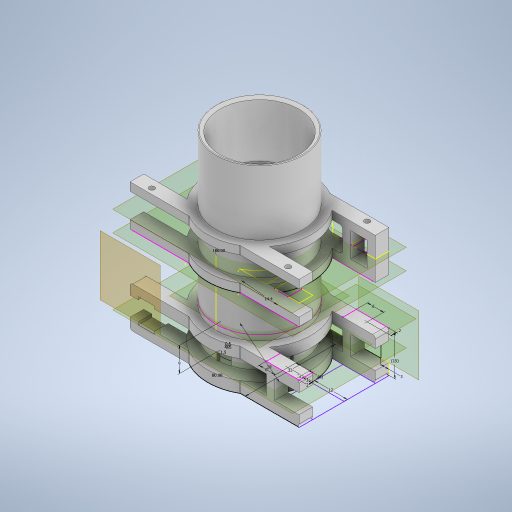
# Autodesk Inventor part: 다단로켓벨브1_ver3
Saved by Autodesk Inventor 2023 (Build 270158000, 158)
## iProperties
Created: 2023-08-24
Part Number: 다단로켓벨브1_ver3
Material: 일반
Document SubType Name: Modeling
Designer: rlatk
Density: 1 g/cm^3
Appearance: 기본값
Author: rlatk
Autodesk Inventor part; units mm, degrees
ref_plane "YZ Plane" through (0, 0, 0) normal (1, 0, 0) x (0, 1, 0)
ref_plane "XZ Plane" through (0, 0, 0) normal (0, 1, 0) x (-1, 0, 0)
ref_plane "XY Plane" through (0, 0, 0) normal (0, 0, 1) x (1, 0, 0)
sketch "스케치1" plane through (0, 0, 0) normal (0, 1, 0) x (-1, 0, 0)
  circle A0 centre (0, 0) radius 14
  circle A1 centre (0, 0) radius 16
  circle A2 centre (0, 0) radius 19
  line L0 (-9.4207, 16.5) -> (-9.4207, -16.5)
  line L1 (-19, 0) -> (-31, 0)
  line L2 (-9.4207, 16.5) -> (-31, 16.5)
  line L3 (-31, 11.5) -> (-9.4207, 11.5)
  line L4 (-9.4207, 11.5) -> (-9.4207, 16.5)
  line L5 (-9.4207, -16.5) -> (-31, -16.5)
  line L6 (-31, -11.5) -> (-9.4207, -11.5)
  line L7 (-31, 0) -> (-31, 16.5)
  line L8 (-31, 0) -> (-31, -16.5)
  line L9 (-19, -16.5) -> (-19, 16.5)
  point P0 (-15.1245, -11.5)
  point P1 (-15.1245, 11.5)
  point P2 (-9.4207, -11.5)
  point P3 (-9.4207, 11.5)
  point P4 (-19, 11.5)
  point P5 (-19, -11.5)
  dimension "d0" = 28
  dimension "d1" = 2
  dimension "d26" = 3
  dimension "d51" = 33
  dimension "d53" = 12
  constraints: 20 end point, 5 point on line, 3 centre point, 3 point on circle, 2 horizontal, 2 perpendicular, 1 coincident, 1 parallel, 1 symmetric about line, 1 vertical
  measures "d0" diameter of A0
  measures "d1" radial gap between concentric circles of A0 A1
  measures "d26" radial gap between concentric circles of A1 A2
  measures "d51" distance of L0.start L0.end
  measures "d53" distance of L1.start L1.end
extrude "돌출1" add sketch "스케치1" along normal blind 39 contours A0 L0 A1 | A0 L0 L6 A1 L3 | L3 A1 L0 | L0 A1 L6
sketch "스케치2" plane through (0, 0, 0) normal (0, 1, 0) x (-1, 0, 0)
  point P0 (0, 0)
ref_plane "작업 평면1" through (0, 18, 0) normal (0, -1, 0) x (1, 0, 0)
sketch "스케치3" plane through (0, 39, 0) normal (0, 1, 0) x (1, 0, 0)
  point P0 (0, 0)
sketch "스케치4" plane through (0, 18, 0) normal (0, -1, 0) x (1, 0, 0)
  circle A0 centre (0, 0) radius 14 projected
  circle A1 centre (0, 0) radius 14
  circle A2 centre (0, 0) radius 3.85
  dimension "d5" = 7.7
  constraints: 2 centre point, 2 coincident, 1 concentric
  measures "d5" diameter of A2
extrude "돌출2" add sketch "스케치4" along normal blind 1 and the other way blind 1
sketch "스케치5" plane through (0, 0, 0) normal (1, 0, 0) x (0, 1, 0)
  line L0 (17, 14) -> (0, 14) projected
  line L1 (0, 14) -> (0, -14) projected
  line L2 (17, -14) -> (17, 14) projected
  line L3 (17, -14) -> (0, -14) projected
  line L4 (8.75, 14) -> (7.25, 14)
  line L5 (7.25, 14) -> (7.25, 12.5)
  line L6 (7.25, 12.5) -> (8.75, 12.5)
  line L7 (8.75, 12.5) -> (8.75, 14)
  line L8 (8.75, 14) -> (8.25, 12.5)
  line L9 (7.25, 13.9506) -> (7.75, 12.5)
  line L10 (0, 16) -> (39, 16) projected
  line L11 (0, -16) -> (0, 16) projected
  line L12 (0, -16) -> (39, -16) projected
  line L13 (0, 16) -> (0.3527, 14)
  line L14 (17, 14) -> (0, 14) projected
  line L15 (0, 16) -> (2.0309, 16) construction
  line L16 (0, 16) -> (0, 14)
  line L17 (0.3527, 14) -> (0, 14)
  line L18 (-8.2062, 0) -> (49.237, 0) projected
  line L19 (39, -16) -> (39, 16) projected
  line L20 (39, -16) -> (39, 16) projected
  line L21 (0, -16) -> (0, 16) projected
  line L22 (39, 14) -> (19, 14) projected
  line L23 (39, -14) -> (19, -14) projected
  line L24 (39, 16) -> (39, 14)
  line L25 (39, 16) -> (38.6473, 14)
  line L26 (39, 14) -> (19, 14) projected
  line L27 (39, 16) -> (41.0309, 16) construction
  line L28 (38.6473, 14) -> (39, 14)
  line L29 (39, 13) -> (19, 13) projected
  point P0 (0, 0)
  point P1 (8.75, 13.25)
  point P2 (8, 14)
  dimension "d10" = 1.5
  dimension "d11" = 1.5
  dimension "d13" = 9
  dimension "d14" = 0.5
  dimension "d15" = 0.5
  dimension "d24" = 80
  dimension "d32" = 100
  constraints: 28 end point, 6 point on line, 4 horizontal, 3 collinear, 2 equal length, 2 midpoint, 2 parallel, 1 perpendicular, 1 other
  measures "d10" distance of L6.end L5.end
  measures "d11" distance of L5.end L4.end
  measures "d13" distance from line of L2 point (8, 14)
  measures "d14" distance of L8.end L6.end
  measures "d15" distance of L5.end L9.end
  measures "d24" angle of L13 L15
  measures "d32" angle of L25 L27
coil "코일1" sketch "스케치5" operation add axis through (0, -10, 0) along (0, 1, 0) pitch 3 turns 2 hand right contours L8 L6 L9 L5 L0
revolve "회전1" cut sketch "스케치5" angle 360 about axis through (0, -10, 0) along (0, 1, 0) contours L0 L11 L13
extrude "돌출3" add sketch "스케치1" along normal blind 4 contours L0 A2 A1 | A1 L3 A2 L0 | A1 L6 A2 L3 | L0 A2 L6 A1
sketch "스케치6" plane through (0, 0, 0) normal (1, 0, 0) x (0, 1, 0)
  line L0 (4, -19) -> (4, 19) projected
  line L1 (4, 19) -> (5.7321, 16)
  line L2 (4, 16) -> (39, 16) projected
  line L3 (4, 19) -> (7.4641, 19) construction
  line L4 (5.7321, 16) -> (4, 16)
  line L5 (4, 16) -> (4, 19)
  line L6 (-7.8, 0) -> (46.8, 0) projected
  point P0 (0, 0)
  dimension "d29" = 60
  constraints: 8 end point, 2 point on line, 1 equal length, 1 horizontal, 1 perpendicular
  measures "d29" angle of L1 L3
revolve "회전2" add sketch "스케치6" angle 360 about axis through (0, -10, 0) along (0, 1, 0)
sketch "스케치7" plane through (0, 0, 0) normal (1, 0, 0) x (0, 1, 0)
  line L0 (6.3094, 16) -> (6.3094, -16) projected
  line L1 (6.3094, 16) -> (11.3094, 16)
  line L2 (5.7321, 16) -> (39, 16) projected
  line L3 (11.3094, 16) -> (6.1446, 14.6071)
  line L4 (6.1446, 14.6071) -> (2.1446, 14.6071)
  line L5 (2.1446, 14.6071) -> (0, 16)
  line L6 (0, 16) -> (0.3527, 14) projected
  line L7 (6.3094, 16) -> (2.3094, 16)
  line L8 (2.3094, 16) -> (0, 17.5)
  line L9 (0, -18) -> (0, 18) projected
  arc A0 (6.1446, 14.6071) -> (11.3094, 16) centre (6.2179, 24.6068) ccw
  arc A1 (0, 16) -> (2.1446, 14.6071) centre (3.1368, 18.482) ccw
  arc A2 (0, 17.5) -> (2.3094, 16) centre (3.2004, 19.8995) ccw
  line L10 (-7.9598, 0) -> (46.8266, 0) projected
  point P0 (0, 0)
  point P1 (6.3094, 14.6515)
  point P2 (6.3094, 14.6072)
  dimension "d35" = 5
  dimension "d36" = 4
  dimension "d37" = 1.5
  dimension "d38" = 10
  dimension "d39" = 4
  dimension "d40" = 4
  constraints: 12 end point, 6 point on circle, 5 point on line, 3 centre point, 2 parallel, 1 other
  measures "d35" distance of L1.start L1.end
  measures "d36" distance of L3.end L4.end
  measures "d37" distance of L8.end L5.end
  measures "d38" radius of A0
  measures "d39" radius of A1
  measures "d40" radius of A2
revolve "회전4" cut sketch "스케치7" angle 18 about axis through (0, -10, 0) along (0, 1, 0) picked at (9.1173, 15.2988) contours L1 L3 L0 | L0 L3 L4 L5 L9 A2 L7 L2 | L3 A0 L0 | A1 L5
pattern_circular "원형 패턴1" count 6 over 360 about axis through (0, -10, 0) along (0, 1, 0) of "회전4"
fillet "모깎기3" radius 1 1 edges at (14, 17, 0)
sketch "스케치8" plane through (0, 17, 0) normal (0, -1, 0) x (1, 0, 0)
  circle A0 centre (0, 0) radius 16 projected
  circle A1 centre (0, 0) radius 15.5305 projected
sketch "스케치9" plane through (0, 19, 0) normal (0, 1, 0) x (1, 0, 0)
  circle A0 centre (0, 0) radius 14.5
  circle A1 centre (0, 0) radius 14
  dimension "d46" = 29
  dimension "d47" = 28
  constraints: 2 centre point, 2 coincident
  measures "d46" diameter of A0
  measures "d47" diameter of A1
extrude "돌출4" cut sketch "스케치9" along normal blind 39 contours A0 | A1
extrude "돌출6" add sketch "스케치1" along normal blind 4 contours A2 L3 L9 L2 | L5 L9 L6 A2 | L9 L3 L7 L2 | L5 L8 L6 L9
sketch "스케치10" plane through (31, 0, -16.5) normal (0, 0, -1) x (-1, 0, 0)
  line L0 (0, 0) -> (21.5793, 0) projected
  line L1 (21.5793, 4) -> (21.5793, 0) projected
  line L2 (0, 4) -> (21.5793, 4) projected
  line L3 (0, 0) -> (0, 4) projected
  line L4 (12, 4) -> (12, 15) projected
  line L5 (12, 4) -> (3, 4)
  line L6 (3, 4) -> (3, 12)
  line L7 (3, 12) -> (12, 12)
  line L8 (12, 12) -> (12, 4)
  point P0 (31, 0)
  dimension "d62" = 3
  constraints: 8 end point, 2 parallel, 1 horizontal, 1 perpendicular
  measures "d62" distance between parallel lines of L3 L6
ref_plane "작업 평면5" through (0, 15, 0) normal (0, 1, 0) x (1, 0, 0)
sketch "스케치11" plane through (0, 15, 0) normal (0, 1, 0) x (1, 0, 0)
  line L0 (31, 16.5) -> (19, 16.5) projected
  line L1 (19, 16.5) -> (19, 11.5) projected
  line L2 (19, -16.5) -> (31, -16.5) projected
  line L3 (19, -11.5) -> (19, -16.5) projected
  line L4 (31, -16.5) -> (31, -11.5) projected
  point P0 (0, 0)
  point P1 (25, 14.5)
  point P2 (25, -14.5)
  dimension "d65" = 2
  dimension "d66" = 6
  dimension "d67" = 2
  dimension "d68" = 6
  dimension "d127" = 6
  measures "d65" distance from line of L0 point (25, 14.5)
  measures "d66" distance from line of L1 point (25, 14.5)
  measures "d67" distance from line of L2 point (25, -14.5)
  measures "d68" distance from line of L3 point (25, -14.5)
  measures "d127" distance from line of point (25, -14.5) L4
ref_plane "작업 평면6" through (19, 12, -16.5) normal (0, -1, 0) x (1, 0, 0)
sketch "스케치12" plane through (19, 12, -16.5) normal (0, -1, 0) x (1, 0, 0)
  line L0 (-3.8755, 5) -> (12, 5) projected
  line L1 (12, 0) -> (-9.5793, 0) projected
  line L2 (12, 5) -> (12, 0) projected
  line L3 (0, 0) -> (0, 5) projected
  line L4 (9, 0) -> (0, 0) projected
  line L5 (0, 5) -> (3, 5)
  line L6 (3, 5) -> (3, 0)
  line L7 (3, 0) -> (0, 0)
  line L8 (0, 0) -> (0, 5)
  line L9 (-9.5793, 33) -> (12, 33) projected
  arc A0 (-9.5793, 33) -> (-9.5793, 0) centre (-19, 16.5) ccw projected
  arc A1 (-3.8755, 5) -> (-3.8755, 28) centre (-19, 16.5) ccw projected
  line L10 (12, 28) -> (-3.8755, 28) projected
  line L11 (12, 33) -> (12, 28) projected
  point P0 (3, 0)
  point P1 (3, 5)
  dimension "d76" = 3
  constraints: 8 end point, 2 parallel, 1 horizontal, 1 perpendicular, 1 point on line
  measures "d76" distance of L6.end L7.end
extrude "돌출9" add sketch "스케치12" along normal blind 12 contours L0 L6 L1 L3
ref_plane "작업 평면7" through (0, 15, 0) normal (0, 1, 0) x (1, 0, 0)
sketch "스케치13" plane through (0, 15, 0) normal (0, 1, 0) x (1, 0, 0)
  circle A0 centre (25, -14.5) radius 1.0065 projected
  line L0 (19, -16.5) -> (31, -16.5) projected
  line L1 (31, -16.5) -> (31, -11.5) projected
  line L2 (31, -11.5) -> (19, -11.5) projected
  line L3 (19, -11.5) -> (19, -16.5) projected
  line L4 (28, -11.5) -> (19, -11.5) projected
  line L5 (19, -16.5) -> (22, -16.5)
  line L6 (22, -16.5) -> (22, -11.5)
  line L7 (22, -11.5) -> (19, -11.5)
  line L8 (19, -11.5) -> (19, -16.5)
  point P0 (0, 0)
  point P1 (22, -11.5)
  dimension "d79" = 3
  constraints: 8 end point, 2 parallel, 1 horizontal, 1 perpendicular, 1 point on line
  measures "d79" distance of L7.end L6.end
extrude "돌출10" add sketch "스케치13" against normal blind 12 contours L3 L2 L6 L0
mirror "미러1" about plane through (0, 0, 0) normal (1, 0, 0) of "돌출6"
ref_plane "작업 평면8" through (-31, 15, 16.5) normal (0, 0, 1) x (1, 0, 0)
sketch "스케치14" plane through (-31, 15, 16.5) normal (0, 0, 1) x (1, 0, 0)
  point P0 (31, -15)
ref_plane "작업 평면9" through (-31, 15, 16.5) normal (0, 0, 1) x (1, 0, 0)
sketch "스케치15" plane through (-31, 15, 16.5) normal (0, 0, 1) x (1, 0, 0)
  line L0 (21.5793, -15) -> (0, -15) projected
  line L1 (21.5793, -11) -> (21.5793, -15) projected
  line L2 (21.5793, -11) -> (0, -11) projected
  line L3 (0, -15) -> (0, -11) projected
  line L4 (3, -3) -> (9, -3)
  line L5 (9, -3) -> (9, -12)
  line L6 (9, -12) -> (3, -12)
  line L7 (3, -12) -> (3, -3)
  point P0 (31, -15)
  point P1 (3, -7.5)
  dimension "d84" = 3
  dimension "d86" = 3
  constraints: 8 end point, 2 parallel, 1 horizontal, 1 midpoint, 1 perpendicular
  measures "d84" distance between parallel lines of L0 L6
  measures "d86" distance from line of L3 point (3, -7.5)
extrude "돌출11" cut sketch "스케치15" against normal blind 33 contours L5 L6 L7 L2 | L2 L7 L4 L5
fillet "모깎기6" radius 1 8 edges at (9.4207, 2, -16.5) (-9.4207, 2, -16.5) (31, 0, -14) (31, 0, 14) (-31, 0, -14) (9.4207, 2, 16.5) (-31, 0, 14) (-9.4207, 2, 16.5)
sketch "스케치17" plane through (0, 39, 0) normal (0, 1, 0) x (1, 0, 0)
  circle A0 centre (0, 0) radius 14.5
  circle A1 centre (0, 0) radius 14.5 projected
  arc A2 (-10.7061, -11.8903) -> (0, -16) centre (0, 0) ccw projected
  circle A3 centre (0, 0) radius 16
  point P0 (-10.7061, -11.8903)
  constraints: 2 coincident, 1 centre point, 3 other
extrude "돌출13" add sketch "스케치17" along normal blind 32
sketch "스케치18" plane through (0, 19, 0) normal (0, 1, 0) x (1, 0, 0)
  circle A0 centre (0, 0) radius 3.85
  circle A1 centre (0, 0) radius 14.5
  constraints: 2 centre point, 2 coincident
sketch "스케치19" plane through (0, 19, 0) normal (0, 1, 0) x (1, 0, 0)
  circle A0 centre (0, 0) radius 7.2
  dimension "d97" = 14.4
  constraints: 1 centre point, 1 coincident
  measures "d97" diameter of A0
sketch "스케치20" plane through (0, 19, 0) normal (0, 1, 0) x (1, 0, 0)
  circle A0 centre (0, 0) radius 8.65
  dimension "d98" = 17.3
  constraints: 1 centre point, 1 coincident
  measures "d98" diameter of A0
extrude "돌출14" add sketch "스케치20" along normal blind 12
extrude "돌출15" cut sketch "스케치18" along normal blind 12 contours A0
sketch "스케치21" plane through (0, 0, 0) normal (0, 0, 1) x (1, 0, 0)
  line L0 (8.65, 31) -> (-8.65, 31) projected
  line L1 (-8.65, 19) -> (8.65, 19) projected
  line L2 (3.85, 17) -> (3.85, 31) projected
  line L3 (8.65, 19) -> (8.65, 31) projected
  line L4 (3.85, 19) -> (8.65, 31)
  line L5 (-8.65, 19) -> (8.65, 19) projected
  line L6 (3.85, 19) -> (8.65, 19)
  line L7 (8.65, 31) -> (-8.65, 31) projected
  line L8 (8.65, 19) -> (8.65, 31)
  line L9 (-3.85, 31) -> (3.85, 31) projected
  line L10 (3.85, 19) -> (3.85, 31)
  line L11 (3.85, 31) -> (8.65, 31)
  point P0 (0, 0)
  constraints: 10 end point, 4 point on line, 2 perpendicular, 1 horizontal
revolve "회전5" cut sketch "스케치21" angle 360 about axis through (0, -10, 0) along (0, 1, 0) contours L4 L2 L0
sketch "스케치22" plane through (0, 19, 0) normal (0, 1, 0) x (1, 0, 0)
  circle A0 centre (0, 0) radius 7.2 projected
  circle A1 centre (0, 0) radius 3.85 projected
  circle A2 centre (0, 0) radius 3.85 projected
  circle A3 centre (0, 0) radius 13 projected
  arc A4 (4.9443, -15.2169) -> (13.8564, -8) centre (0, 0) ccw projected
  arc A5 (0, -16) -> (4.9443, -15.2169) centre (0, 0) ccw projected
  arc A6 (-10.7061, -11.8903) -> (0, -16) centre (0, 0) ccw projected
  arc A7 (-13.8564, -8) -> (-10.7061, -11.8903) centre (0, 0) ccw projected
  arc A8 (-15.6504, 3.3266) -> (-13.8564, -8) centre (0, 0) ccw projected
  arc A9 (-13.8564, 8) -> (-15.6504, 3.3266) centre (0, 0) ccw projected
  arc A10 (-4.9443, 15.2169) -> (-13.8564, 8) centre (0, 0) ccw projected
  arc A11 (0, 16) -> (-4.9443, 15.2169) centre (0, 0) ccw projected
  arc A12 (10.7061, 11.8903) -> (0, 16) centre (0, 0) ccw projected
  arc A13 (13.8564, 8) -> (10.7061, 11.8903) centre (0, 0) ccw projected
  arc A14 (15.6504, -3.3266) -> (13.8564, 8) centre (0, 0) ccw projected
  arc A15 (13.8564, -8) -> (15.6504, -3.3266) centre (0, 0) ccw projected
  circle A16 centre (0, 0) radius 14 projected
  circle A17 centre (0, 0) radius 7.2
  line L0 (0, -13.9506) -> (0, -12.5) projected
  line L1 (0, 16) -> (0, 14.6072) projected
  circle A18 centre (0, 0) radius 16
  circle A19 centre (0, 0) radius 7.2
  arc A20 (0, 14.6071) -> (-4.5138, 13.8921) centre (0, 0) ccw projected
  circle A21 centre (0, 0) radius 14.6071
  point P0 (-4.5138, 13.8921)
  constraints: 4 coincident, 2 centre point, 2 concentric, 1 vertical alignment, 5 other
extrude "돌출16" add sketch "스케치22" along normal blind 22.5 contours A3 | A16 | A21 A20
sketch "스케치23" plane through (0, 41.5, 0) normal (0, 1, 0) x (1, 0, 0)
  arc A0 (9.1983, 16.625) -> (-9.1983, 16.625) centre (0, 0) ccw projected
  line L0 (0, -11.0274) -> (-9.55, -5.5137)
  line L1 (-9.55, -5.5137) -> (-9.55, 5.5137)
  line L2 (-9.55, 5.5137) -> (0, 11.0274)
  line L3 (0, 11.0274) -> (9.55, 5.5137)
  line L4 (9.55, 5.5137) -> (9.55, -5.5137)
  line L5 (9.55, -5.5137) -> (0, -11.0274)
  circle A1 centre (0, 0) radius 14.5 projected
  circle A2 centre (0, 0) radius 14.5
  dimension "d106" = 19.1
  constraints: 12 end point, 2 coincident, 1 centre point, 13 other
  measures "d106" distance between parallel lines of L0 L3
extrude "돌출17" add sketch "스케치23" along normal blind 9
sketch "스케치24" plane through (0, 0, 0) normal (1, 0, 0) x (0, 1, 0)
  line L0 (71, -16) -> (71, 16) projected
  line L1 (5.7321, 16) -> (71, 16) projected
  line L2 (50.5, 14.5) -> (50.5, -14.5) projected
  line L3 (71, 14.5) -> (71, -14.5) projected
  line L4 (50.5, 14.5) -> (71, 14.5) projected
  line L5 (71, 16) -> (70.134, 14.5)
  line L6 (71, 16) -> (72.7321, 16) construction
  line L7 (70.134, 14.5) -> (71, 14.5)
  line L8 (71, 16) -> (71, 14.5)
  line L9 (-14.5464, 0) -> (87.2785, 0) projected
  point P0 (0, 0)
  dimension "d109" = 120
  constraints: 8 end point, 2 collinear, 1 equal length, 1 horizontal, 1 point on line
  measures "d109" angle of L5 L6
revolve "회전6" cut sketch "스케치24" angle 360 about axis through (0, -10, 0) along (0, 1, 0) contours L4 L5 L0
fillet "모깎기8" radius 0.2 2 edges at (5.7339, 71, -14.9373) (-5.7339, 71, 14.9373)
ref_plane "작업 평면10" through (31, 15, -16.5) normal (0, 0, -1) x (-1, 0, 0)
sketch "스케치25" plane through (31, 15, -16.5) normal (0, 0, -1) x (-1, 0, 0)
  line L0 (1, -15) -> (21.3175, -15) projected
  line L1 (0, 0) -> (12, 0) projected
  point P0 (31, -15)
  dimension "d112" = 15
  measures "d112" distance between parallel lines of L0 L1
ref_plane "작업 평면2" through (0, 7.5, 0) normal (0, -1, 0) x (1, 0, 0)
mirror "미러4" about plane through (0, 7.5, 0) normal (0, -1, 0) of "돌출6", "미러1", "돌출3", "돌출11", "모깎기6", "돌출9", "돌출10"
ref_plane "작업 평면3" through (0, 32, 0) normal (0, -1, 0) x (1, 0, 0)
sketch "스케치26" plane through (0, 32, 0) normal (0, -1, 0) x (1, 0, 0)
  circle A0 centre (0, 0) radius 16 projected
  line L0 (-30, 16.5) -> (-30, 11.5) projected
  line L1 (-9.6825, 16.5) -> (-30, 16.5) projected
  arc A1 (-9.6825, 16.5) -> (-9.1983, 16.625) centre (-9.6825, 17.5) ccw projected
  arc A2 (9.1983, 16.625) -> (-9.1983, 16.625) centre (0, 0) ccw projected
  arc A3 (9.1983, 16.625) -> (9.6825, 16.5) centre (9.6825, 17.5) ccw projected
  line L2 (9.6825, 16.5) -> (30, 16.5) projected
  line L3 (30, 11.5) -> (30, 16.5) projected
  line L4 (30, 11.5) -> (15.1245, 11.5) projected
  arc A4 (15.1245, -11.5) -> (15.1245, 11.5) centre (0, 0) ccw projected
  line L5 (15.1245, -11.5) -> (30, -11.5) projected
  line L6 (30, -16.5) -> (30, -11.5) projected
  line L7 (30, -16.5) -> (9.6825, -16.5) projected
  arc A5 (9.6825, -16.5) -> (9.1983, -16.625) centre (9.6825, -17.5) ccw projected
  arc A6 (-9.1983, -16.625) -> (9.1983, -16.625) centre (0, 0) ccw projected
  arc A7 (-9.1983, -16.625) -> (-9.6825, -16.5) centre (-9.6825, -17.5) ccw projected
  line L8 (-30, -16.5) -> (-9.6825, -16.5) projected
  line L9 (-30, -11.5) -> (-30, -16.5) projected
  line L10 (-15.1245, -11.5) -> (-30, -11.5) projected
  arc A8 (-15.1245, 11.5) -> (-15.1245, -11.5) centre (0, 0) ccw projected
  line L11 (-30, 11.5) -> (-15.1245, 11.5) projected
  circle A9 centre (0, 0) radius 3.85 projected
  circle A10 centre (0, 0) radius 19
  circle A11 centre (0, 0) radius 16
  constraints: 2 centre point, 2 coincident, 1 concentric
sketch "스케치27" plane through (0, 32, 0) normal (0, -1, 0) x (1, 0, 0)
  line L0 (31, 16.5) -> (31, 11.5) projected
  line L1 (31, 11.5) -> (9.4207, 11.5) projected
  line L2 (30, 16.5) -> (31, 16.5) projected
  line L3 (31, 16.5) -> (31, 11.5) projected
  line L4 (31, 11.5) -> (30, 11.5) projected
  line L5 (30, 11.5) -> (30, 16.5) projected
  line L6 (31, -16.5) -> (30, -16.5) projected
  line L7 (30, -16.5) -> (30, -11.5) projected
  line L8 (30, -11.5) -> (31, -11.5) projected
  line L9 (31, -11.5) -> (31, -16.5) projected
  line L10 (-30, -16.5) -> (-31, -16.5) projected
  line L11 (-31, -16.5) -> (-31, -11.5) projected
  line L12 (-31, -11.5) -> (-30, -11.5) projected
  line L13 (-30, -11.5) -> (-30, -16.5) projected
  line L14 (-31, 16.5) -> (-30, 16.5) projected
  line L15 (-30, 16.5) -> (-30, 11.5) projected
  line L16 (-30, 11.5) -> (-31, 11.5) projected
  line L17 (-31, 11.5) -> (-31, 16.5) projected
  arc A0 (-15.1245, 11.5) -> (-15.1245, -11.5) centre (0, 0) ccw projected
  circle A1 centre (0, 0) radius 19 projected
  circle A2 centre (0, 0) radius 16 projected
  circle A3 centre (0, 0) radius 16 projected
  line L18 (-30, 16.5) -> (-30, 11.5) projected
  line L19 (-9.6825, 16.5) -> (-30, 16.5) projected
  arc A4 (-9.6825, 16.5) -> (-9.1983, 16.625) centre (-9.6825, 17.5) ccw projected
  arc A5 (9.1983, 16.625) -> (-9.1983, 16.625) centre (0, 0) ccw projected
  arc A6 (9.1983, 16.625) -> (9.6825, 16.5) centre (9.6825, 17.5) ccw projected
  line L20 (9.6825, 16.5) -> (30, 16.5) projected
  line L21 (30, 11.5) -> (30, 16.5) projected
  line L22 (30, 11.5) -> (15.1245, 11.5) projected
  arc A7 (15.1245, -11.5) -> (15.1245, 11.5) centre (0, 0) ccw projected
  line L23 (15.1245, -11.5) -> (30, -11.5) projected
  line L24 (30, -16.5) -> (30, -11.5) projected
  line L25 (30, -16.5) -> (9.6825, -16.5) projected
  arc A8 (9.6825, -16.5) -> (9.1983, -16.625) centre (9.6825, -17.5) ccw projected
  arc A9 (-9.1983, -16.625) -> (9.1983, -16.625) centre (0, 0) ccw projected
  arc A10 (-9.1983, -16.625) -> (-9.6825, -16.5) centre (-9.6825, -17.5) ccw projected
  line L26 (-30, -16.5) -> (-9.6825, -16.5) projected
  line L27 (-30, -11.5) -> (-30, -16.5) projected
  line L28 (-15.1245, -11.5) -> (-30, -11.5) projected
  arc A11 (-15.1245, 11.5) -> (-15.1245, -11.5) centre (0, 0) ccw projected
  line L29 (-30, 11.5) -> (-15.1245, 11.5) projected
  point P0 (-15.1245, -11.5)
extrude "돌출18" add sketch "스케치27" against normal blind 3
ref_plane "작업 평면4" through (0, 39.5, 0) normal (0, -1, 0) x (1, 0, 0)
mirror "미러5" about plane through (0, 39.5, 0) normal (0, -1, 0) of "돌출18"
sketch "스케치28" plane through (0, 39.5, 0) normal (0, -1, 0) x (1, 0, 0)
  line L0 (27, 11.5) -> (27, 16.5) projected
  line L1 (22, -16.5) -> (27, -16.5) projected
  line L2 (27, -11.5) -> (22, -11.5) projected
  line L3 (28, -16.5) -> (27, -16.5) projected
  line L4 (27, -16.5) -> (27, -11.5) projected
  line L5 (27, -11.5) -> (28, -11.5) projected
  line L6 (28, -11.5) -> (28, -16.5) projected
  line L7 (23, -16.5) -> (22, -16.5) projected
  line L8 (22, -16.5) -> (22, -11.5) projected
  line L9 (22, -11.5) -> (23, -11.5) projected
  line L10 (23, -11.5) -> (23, -16.5) projected
  line L11 (18, -11.5) -> (19, -11.5) projected
  line L12 (19, -11.5) -> (19, -16.5) projected
  line L13 (19, -16.5) -> (18, -16.5) projected
  line L14 (18, -16.5) -> (18, -11.5) projected
  line L15 (19, -16.5) -> (9.6825, -16.5) projected
  arc A0 (9.6825, -16.5) -> (9.1983, -16.625) centre (9.6825, -17.5) ccw projected
  arc A1 (9.1983, -16.625) -> (15.1245, -11.5) centre (0, 0) ccw projected
  line L16 (15.1245, -11.5) -> (19, -11.5) projected
  line L17 (22, -11.5) -> (31, -11.5) projected
  line L18 (31, -11.5) -> (31, -16.5) projected
  line L19 (31, -16.5) -> (22, -16.5) projected
  line L20 (19, 16.5) -> (19, 11.5) projected
  line L21 (19, -11.5) -> (19, -16.5) projected
  line L22 (19, 11.5) -> (15.1245, 11.5) projected
  arc A2 (15.1245, 11.5) -> (9.1983, 16.625) centre (0, 0) ccw projected
  arc A3 (9.1983, 16.625) -> (9.6825, 16.5) centre (9.6825, 17.5) ccw projected
  line L23 (9.6825, 16.5) -> (19, 16.5) projected
  line L24 (22, -16.5) -> (22, -11.5) projected
  line L25 (22, 11.5) -> (27, 11.5) projected
  line L26 (27, 16.5) -> (22, 16.5) projected
  line L27 (22, 16.5) -> (31, 16.5) projected
  line L28 (31, 16.5) -> (31, 11.5) projected
  line L29 (31, 11.5) -> (22, 11.5) projected
  line L30 (27, -16.5) -> (27, -11.5) projected
  line L31 (22, 11.5) -> (22, 16.5) projected
  line L32 (22, -16.5) -> (22, -11.5) projected
  line L33 (22, 11.5) -> (22, 16.5) projected
sketch "스케치29" plane through (0, 39.5, 0) normal (0, -1, 0) x (1, 0, 0)
  point P0 (0, 0)
sketch "스케치30" plane through (0, 39.5, 0) normal (0, -1, 0) x (1, 0, 0)
  line L0 (30, -16.5) -> (9.6825, -16.5) projected
  line L1 (19, -16.5) -> (9.6825, -16.5) projected
  line L2 (31, -11.5) -> (31, -16.5) projected
  line L3 (15.1245, -11.5) -> (31, -11.5) projected
  line L4 (31, 16.5) -> (31, 11.5) projected
  line L5 (31, 11.5) -> (15.1245, 11.5) projected
  arc A0 (15.1245, -11.5) -> (15.1245, 11.5) centre (0, 0) ccw projected
  line L6 (15.1245, -11.5) -> (31, -11.5) projected
  line L7 (31, -11.5) -> (31, -16.5) projected
  line L8 (31, -16.5) -> (9.6825, -16.5) projected
  arc A1 (9.6825, -16.5) -> (9.1983, -16.625) centre (9.6825, -17.5) ccw projected
  arc A2 (-9.1983, -16.625) -> (9.1983, -16.625) centre (0, 0) ccw projected
  arc A3 (-9.1983, -16.625) -> (-9.6825, -16.5) centre (-9.6825, -17.5) ccw projected
  line L9 (-9.6825, -16.5) -> (-31, -16.5) projected
  line L10 (-31, -16.5) -> (-31, -11.5) projected
  line L11 (-31, -11.5) -> (-15.1245, -11.5) projected
  arc A4 (-15.1245, 11.5) -> (-15.1245, -11.5) centre (0, 0) ccw projected
  line L12 (-15.1245, 11.5) -> (-31, 11.5) projected
  line L13 (-31, 11.5) -> (-31, 16.5) projected
  line L14 (-31, 16.5) -> (-9.6825, 16.5) projected
  arc A5 (-9.6825, 16.5) -> (-9.1983, 16.625) centre (-9.6825, 17.5) ccw projected
  arc A6 (9.1983, 16.625) -> (-9.1983, 16.625) centre (0, 0) ccw projected
  arc A7 (9.1983, 16.625) -> (9.6825, 16.5) centre (9.6825, 17.5) ccw projected
  line L15 (9.6825, 16.5) -> (31, 16.5) projected
  circle A8 centre (0, 0) radius 16 projected
  line L16 (-28, -11.5) -> (-27, -11.5) projected
  line L17 (-27, -11.5) -> (-27, -16.5) projected
  line L18 (-27, -16.5) -> (-28, -16.5) projected
  line L19 (-28, -16.5) -> (-28, -11.5) projected
  line L20 (-22, -11.5) -> (-28, -11.5) projected
  line L21 (-28, -16.5) -> (-22, -16.5) projected
  line L22 (-23, -11.5) -> (-22, -11.5) projected
  line L23 (-22, -11.5) -> (-22, -16.5) projected
  line L24 (-22, -16.5) -> (-23, -16.5) projected
  line L25 (-23, -16.5) -> (-23, -11.5) projected
  line L26 (-18, -11.5) -> (-18, -16.5) projected
  line L27 (-19, -11.5) -> (-18, -11.5) projected
  line L28 (-18, -11.5) -> (-18, -16.5) projected
  line L29 (-18, -16.5) -> (-19, -16.5) projected
  line L30 (-19, -16.5) -> (-19, -11.5) projected
  line L31 (-15.1245, -11.5) -> (-22, -11.5) projected
  arc A9 (-15.1245, -11.5) -> (-9.1983, -16.625) centre (0, 0) ccw projected
  arc A10 (-9.1983, -16.625) -> (-9.6825, -16.5) centre (-9.6825, -17.5) ccw projected
  line L32 (-22, -16.5) -> (-9.6825, -16.5) projected
  line L33 (-28, 11.5) -> (-22, 11.5) projected
  line L34 (-22, 16.5) -> (-28, 16.5) projected
  line L35 (-28, 16.5) -> (-27, 16.5) projected
  line L36 (-27, 16.5) -> (-27, 11.5) projected
  line L37 (-27, 11.5) -> (-28, 11.5) projected
  line L38 (-28, 11.5) -> (-28, 16.5) projected
  line L39 (-23, 16.5) -> (-22, 16.5) projected
  line L40 (-22, 16.5) -> (-22, 11.5) projected
  line L41 (-22, 11.5) -> (-23, 11.5) projected
  line L42 (-23, 11.5) -> (-23, 16.5) projected
  line L43 (-19, 16.5) -> (-18, 16.5) projected
  line L44 (-18, 16.5) -> (-18, 11.5) projected
  line L45 (-18, 11.5) -> (-19, 11.5) projected
  line L46 (-19, 11.5) -> (-19, 16.5) projected
  line L47 (-9.6825, 16.5) -> (-22, 16.5) projected
  arc A11 (-9.6825, 16.5) -> (-9.1983, 16.625) centre (-9.6825, 17.5) ccw projected
  arc A12 (-9.1983, 16.625) -> (-15.1245, 11.5) centre (0, 0) ccw projected
  line L48 (-22, 11.5) -> (-15.1245, 11.5) projected
  line L49 (27, 11.5) -> (27, 16.5) projected
  line L50 (22, 11.5) -> (27, 11.5) projected
  line L51 (27, 16.5) -> (22, 16.5) projected
  line L52 (23, 11.5) -> (22, 11.5) projected
  line L53 (22, 11.5) -> (22, 16.5) projected
  line L54 (22, 16.5) -> (23, 16.5) projected
  line L55 (23, 16.5) -> (23, 11.5) projected
  line L56 (28, 11.5) -> (27, 11.5) projected
  line L57 (27, 11.5) -> (27, 16.5) projected
  line L58 (27, 16.5) -> (28, 16.5) projected
  line L59 (18, 16.5) -> (19, 16.5) projected
  line L60 (19, 16.5) -> (19, 11.5) projected
  line L61 (19, 11.5) -> (18, 11.5) projected
  line L62 (18, 11.5) -> (18, 16.5) projected
  line L63 (19, 11.5) -> (15.1245, 11.5) projected
  arc A13 (15.1245, 11.5) -> (9.1983, 16.625) centre (0, 0) ccw projected
  arc A14 (9.1983, 16.625) -> (9.6825, 16.5) centre (9.6825, 17.5) ccw projected
  line L64 (9.6825, 16.5) -> (19, 16.5) projected
  line L65 (22, 16.5) -> (31, 16.5) projected
  line L66 (31, 16.5) -> (31, 11.5) projected
  line L67 (31, 11.5) -> (22, 11.5) projected
  line L68 (19, 16.5) -> (19, 11.5) projected
  line L69 (28, 11.5) -> (28, 16.5) projected
  line L70 (-31, 16.5) -> (-31, 11.5) projected
  line L71 (-31, -11.5) -> (-31, -16.5) projected
  line L72 (31, -16.5) -> (22, -16.5) projected
  line L73 (30, -16.5) -> (31, -16.5) projected
  line L74 (-22, 11.5) -> (-22, 16.5) projected
  line L75 (-28, 16.5) -> (-28, 11.5) projected
  line L76 (-31, 11.5) -> (-28, 11.5) projected
  line L77 (-28, 16.5) -> (-31, 16.5) projected
  line L78 (-28, 16.5) -> (-28, 11.5) projected
  line L79 (-22, 16.5) -> (-22, 11.5) projected
  line L80 (-22, -16.5) -> (-22, -11.5) projected
  line L81 (-28, -11.5) -> (-28, -16.5) projected
  line L82 (-31, -16.5) -> (-28, -16.5) projected
  line L83 (-28, -11.5) -> (-31, -11.5) projected
  line L84 (-22, -11.5) -> (-22, -16.5) projected
  line L85 (-28, -11.5) -> (-28, -16.5) projected
  line L86 (31, -16.5) -> (30, -16.5) projected
  line L87 (31, -16.5) -> (22, -16.5) projected
  line L88 (19, -16.5) -> (9.6825, -16.5) projected
  line L89 (30, -16.5) -> (9.6825, -16.5) projected
  line L90 (22, 11.5) -> (22, 16.5) projected
  line L91 (22, 11.5) -> (22, 16.5) projected
sketch "스케치31" plane through (0, 39.5, 0) normal (0, -1, 0) x (1, 0, 0)
  line L0 (9.6825, 16.5) -> (31, 16.5) projected
  line L1 (31, 16.5) -> (31, 11.5) projected
  line L2 (31, 11.5) -> (15.1245, 11.5) projected
  line L3 (28, 16.5) -> (28, 11.5) projected
  line L4 (15.1245, -11.5) -> (31, -11.5) projected
  line L5 (31, -11.5) -> (31, -16.5) projected
  line L6 (31, -16.5) -> (9.6825, -16.5) projected
  line L7 (28, -11.5) -> (28, -16.5) projected
  line L8 (22, -16.5) -> (22, -11.5) projected
  line L9 (-31, -11.5) -> (-15.1245, -11.5) projected
  line L10 (-9.6825, -16.5) -> (-31, -16.5) projected
  line L11 (-31, -16.5) -> (-31, -11.5) projected
  line L12 (-28, -16.5) -> (-28, -11.5) projected
  line L13 (-22, -11.5) -> (-22, -16.5) projected
  line L14 (-19, -16.5) -> (-19, -11.5) projected
  line L15 (-19, 11.5) -> (-19, 16.5) projected
  line L16 (-22, 16.5) -> (-22, 11.5) projected
  line L17 (-28, 11.5) -> (-28, 16.5) projected
  line L18 (-31, 16.5) -> (-9.6825, 16.5) projected
  line L19 (-15.1245, 11.5) -> (-31, 11.5) projected
  line L20 (-31, 11.5) -> (-31, 16.5) projected
  line L21 (-28, 16.5) -> (-31, 16.5)
  line L22 (-31, 16.5) -> (-31, 11.5)
  line L23 (-31, 11.5) -> (-28, 11.5)
  line L24 (-28, 11.5) -> (-28, 16.5)
  line L25 (-28, -11.5) -> (-31, -11.5)
  line L26 (-31, -11.5) -> (-31, -16.5)
  line L27 (-31, -16.5) -> (-28, -16.5)
  line L28 (-28, -16.5) -> (-28, -11.5)
  line L29 (31, -11.5) -> (28, -11.5)
  line L30 (28, -11.5) -> (28, -16.5)
  line L31 (28, -16.5) -> (31, -16.5)
  line L32 (31, -16.5) -> (31, -11.5)
  line L33 (31, 16.5) -> (28, 16.5)
  line L34 (28, 16.5) -> (28, 11.5)
  line L35 (28, 11.5) -> (31, 11.5)
  line L36 (31, 11.5) -> (31, 16.5)
  line L37 (22, 11.5) -> (22, 16.5) projected
  line L38 (19, 16.5) -> (19, 11.5) projected
  line L39 (22, 16.5) -> (19, 16.5)
  line L40 (19, 16.5) -> (19, 11.5)
  line L41 (19, 11.5) -> (22, 11.5)
  line L42 (22, 11.5) -> (22, 16.5)
  line L43 (22, -11.5) -> (19, -11.5)
  line L44 (19, -11.5) -> (19, -16.5)
  line L45 (19, -16.5) -> (22, -16.5)
  line L46 (22, -16.5) -> (22, -11.5)
  line L47 (-19, 11.5) -> (-19, 16.5) projected
  line L48 (-19, 16.5) -> (-22, 16.5)
  line L49 (-22, 16.5) -> (-22, 11.5)
  line L50 (-22, 11.5) -> (-19, 11.5)
  line L51 (-19, 11.5) -> (-19, 16.5)
  line L52 (-19, -11.5) -> (-22, -11.5)
  line L53 (-22, -11.5) -> (-22, -16.5)
  line L54 (-22, -16.5) -> (-19, -16.5)
  line L55 (-19, -16.5) -> (-19, -11.5)
  point P0 (0, 0)
  point P1 (-23, 11.5)
  constraints: 64 end point, 16 parallel, 8 horizontal, 8 perpendicular, 2 point on line
extrude "돌출19" [suppressed]
extrude "돌출20" add sketch "스케치31" along normal blind 7.5 and the other way blind 5 contours L4 L8 L6 L44 | L4 L5 L6 L7
sketch "스케치32" plane through (9.6825, 47, 16.5) normal (0, 1, 0) x (1, 0, 0)
  point P0 (-9.6825, 16.5)
sketch "스케치33" plane through (9.6825, 47, 16.5) normal (0, 1, 0) x (1, 0, 0)
  point P0 (-9.6825, 16.5)
sketch "스케치34" plane through (9.6825, 47, 16.5) normal (0, 1, 0) x (1, 0, 0)
  line L0 (21.3175, 0) -> (0, 0) projected
  line L1 (21.3175, 5) -> (21.3175, 0) projected
  line L2 (0, 33) -> (21.3175, 33) projected
  line L3 (21.3175, 33) -> (21.3175, 28) projected
  line L4 (-40.6825, 33) -> (-19.3649, 33) projected
  line L5 (-40.6825, 28) -> (-40.6825, 33) projected
  line L6 (-19.3649, 0) -> (-40.6825, 0) projected
  line L7 (-40.6825, 0) -> (-40.6825, 5) projected
  point P0 (-9.6825, 16.5)
  point P1 (15.3175, 2)
  point P2 (15.3175, 31)
  point P3 (-34.6825, 31)
  point P4 (-34.6825, 2)
  dimension "d128" = 2
  dimension "d129" = 6
  dimension "d130" = 2
  dimension "d131" = 6
  dimension "d132" = 2
  dimension "d133" = 6
  dimension "d134" = 2
  dimension "d135" = 6
  measures "d128" distance from line of point (15.318, 2) L0
  measures "d129" distance from line of L1 point (15.318, 2)
  measures "d130" distance from line of L2 point (15.318, 31)
  measures "d131" distance from line of L3 point (15.318, 31)
  measures "d132" distance from line of L4 point (-34.682, 31)
  measures "d133" distance from line of L5 point (-34.682, 31)
  measures "d134" distance from line of L6 point (-34.682, 2)
  measures "d135" distance from line of L7 point (-34.682, 2)
fillet "모깎기10" radius 1 2 edges at (19, 35, -14) (19, 44, -14)
hole "구멍3" at (25, 47, 14.5) at (25, 47, -14.5) at (-25, 47, -14.5) at (-25, 47, 14.5) direction (0, -1, 0) diameter 2 depth 6.3 tip angle 118
